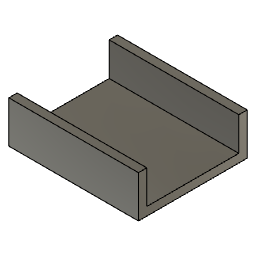
generic luos module holder v1 (Autodesk Fusion 360 design; units mm, degrees)
Autodesk Fusion 360 part; units mm, degrees
note: some values were not read from the file. Set by a fixed rule: which face or edge a step refers to.
sketch "Sketch1" plane through (0, 0, 0) normal (0, 0, 1) x (1, 0, 0)
  line L0 (0, 0) -> (31, 0)
  line L1 (31, 0) -> (31, 26)
  line L2 (31, 26) -> (0, 26)
  line L3 (0, 26) -> (0, 0)
  dimension "d1" = 31
  dimension "d2" = 26
  constraint horizontal L0
  constraint vertical L1
  constraint horizontal L2
  constraint vertical L3
  constraint coincident L0.start L3.end
  measures "d1" distance of L0.start L0.end
  measures "d2" distance of L0.start L2.end
extrude "Extrude1" add sketch "Sketch1" along normal blind 10
shell "Shell1" thickness 2 removed faces 1 at (10.3333, 17.3333, 10)
extrude "Extrude2" cut 1 faces at (2, 16.6667, 4.6667) along direction (-1, 0, 0) blind 10
extrude "Extrude3" cut 1 faces at (29, 16.6667, 7.3333) along direction (1, 0, 0) blind 20
